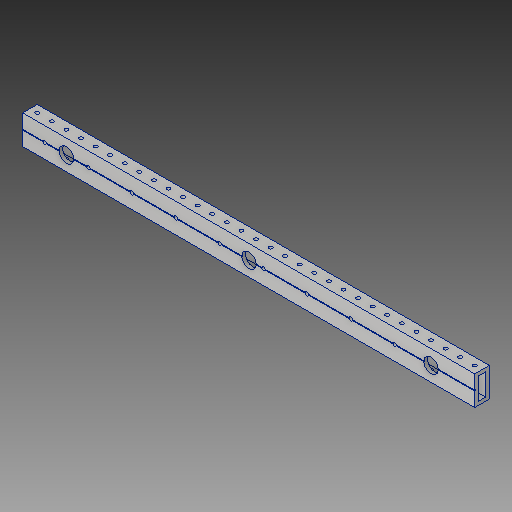
# Autodesk Inventor part: 2AM-17-01-Side Frame
Saved by Autodesk Inventor 2017 (Build 210142000, 142)
## iProperties
Created: 2017-12-28
Part Number: 2AM-17-01-Side Frame
Material: Aluminum 6061
Document SubType Name: Modeling
Designer: anikasoojin
Density: 2.7 g/cm^3
Appearance: Aluminum - Flat
Mass: 1616.08 g
Surface Area: 2052.62 cm^2
Volume: 598.55 cm^3
Author: anikasoojin
Autodesk Inventor part; units mm, degrees
ref_plane "YZ Plane" through (0, 0, 0) normal (1, 0, 0) x (0, 1, 0)
ref_plane "XZ Plane" through (0, 0, 0) normal (0, 1, 0) x (-1, 0, 0)
ref_plane "XY Plane" through (0, 0, 0) normal (0, 0, 1) x (1, 0, 0)
sketch "Sketch1" plane through (0, 0, 0) normal (1, 0, 0) x (0, 1, 0)
  line L0 (5.2493, 16.002) -> (-45.5507, 16.002)
  line L1 (-45.5507, 16.002) -> (-45.5507, -9.398)
  line L2 (-45.5507, -9.398) -> (5.2493, -9.398)
  line L3 (5.2493, -9.398) -> (5.2493, 16.002)
  line L4 (-1.1007, 9.652) -> (-39.2007, 9.652)
  line L5 (-39.2007, 9.652) -> (-39.2007, -3.048)
  line L6 (-39.2007, -3.048) -> (-1.1007, -3.048)
  line L7 (-1.1007, -3.048) -> (-1.1007, 9.652)
  point P0 (0, 0)
  dimension "d0" = 25.4
  dimension "d1" = 50.8
  dimension "d2" = 6.35
  constraints: 16 end point, 4 parallel, 2 perpendicular, 1 horizontal, 3 other
  measures "d0" distance of L2.end L0.start
  measures "d1" distance of L1.end L2.end
  measures "d2" distance between parallel lines of L3 L7
extrude "Extrusion1" add sketch "Sketch1" along normal blind 787.4
sketch "Sketch2" plane through (0, -45.5507, 16.002) normal (0, 0, 1) x (1, 0, 0)
  line L0 (0, 50.8) -> (0, 0) projected
  line L1 (0, 25.4) -> (787.4, 25.4) construction
  line L2 (787.4, 50.8) -> (787.4, 0) projected
  line L3 (0, 50.8) -> (787.4, 50.8) projected
  line L4 (393.7, 50.8) -> (394.6973, 0) construction
  line L5 (0, 0) -> (787.4, 0) projected
  circle A0 centre (394.1986, 25.4) radius 12.7
  circle A1 centre (711.2, 25.4) radius 12.7
  circle A2 centre (76.2, 25.4) radius 12.7
  circle A3 centre (38.1, 25.4) radius 3.175
  circle A4 centre (114.3, 25.4) radius 3.175
  circle A5 centre (190.5, 25.4) radius 3.175
  circle A6 centre (266.7, 25.4) radius 3.175
  circle A7 centre (342.9, 25.4) radius 3.175
  circle A8 centre (419.1, 25.4) radius 3.175
  circle A9 centre (495.3, 25.4) radius 3.175
  circle A10 centre (571.5, 25.4) radius 3.175
  circle A11 centre (647.7, 25.4) radius 3.175
  point P0 (0, 45.5507)
  dimension "d5" = 25.4
  dimension "d6" = 25.4
  dimension "d7" = 76.2
  dimension "d8" = 25.4
  dimension "d9" = 76.2
  dimension "d10" = 6.35
  dimension "d11" = 38.1
  dimension "d14" = 76.2
  constraints: 12 centre point, 4 end point, 4 midpoint, 4 point on line, 1 horizontal, 16 other
  measures "d5" diameter of A0
  measures "d6" diameter of A1
  measures "d7" distance of L1.end A1.centre
  measures "d8" diameter of A2
  measures "d9" distance of L1.start A2.centre
  measures "d10" diameter of A3
  measures "d11" distance of L1.start A3.centre
  measures "d14" distance of A3.centre A4.centre
extrude "Extrusion2" cut sketch "Sketch2" against normal through all contours A0 | A1 | A2 | A3 | A4 | A5 | A6 | A7 | A8 | A9 | A10 | A11
sketch "Sketch3" plane through (0, -45.5507, 16.002) normal (0, 0, 1) x (1, 0, 0)
  line L0 (0, 6.35) -> (0, 44.45) projected
  line L1 (0, 25.4) -> (787.4, 25.4) construction
  line L2 (787.4, 44.45) -> (787.4, 6.35) projected
  line L3 (0, 26.035) -> (787.4, 26.035)
  line L4 (0, 24.765) -> (787.4, 24.765)
  point P0 (0, 45.5507)
  dimension "d21" = 0.635
  dimension "d22" = 0.635
  constraints: 6 end point, 4 point on line, 2 midpoint, 2 parallel
  measures "d21" distance of L3.start L1.start
  measures "d22" distance of L1.start L4.start
extrude "Extrusion3" cut sketch "Sketch3" against normal blind 1.27
sketch "Sketch4" plane through (0, 5.2493, 16.002) normal (0, 1, 0) x (1, 0, 0)
  line L0 (0, 0) -> (0, 25.4) projected
  line L1 (30.4329, 12.7) -> (0, 12.7) construction
  circle A0 centre (12.7, 12.7) radius 3.175
  line L2 (55.8329, 12.7) -> (25.4, 12.7) construction
  circle A1 centre (38.1, 12.7) radius 3.175
  line L3 (81.2329, 12.7) -> (50.8, 12.7) construction
  circle A2 centre (63.5, 12.7) radius 3.175
  line L4 (106.6329, 12.7) -> (76.2, 12.7) construction
  circle A3 centre (88.9, 12.7) radius 3.175
  line L5 (132.0329, 12.7) -> (101.6, 12.7) construction
  circle A4 centre (114.3, 12.7) radius 3.175
  line L6 (157.4329, 12.7) -> (127, 12.7) construction
  circle A5 centre (139.7, 12.7) radius 3.175
  line L7 (182.8329, 12.7) -> (152.4, 12.7) construction
  circle A6 centre (165.1, 12.7) radius 3.175
  line L8 (208.2329, 12.7) -> (177.8, 12.7) construction
  circle A7 centre (190.5, 12.7) radius 3.175
  line L9 (233.6329, 12.7) -> (203.2, 12.7) construction
  circle A8 centre (215.9, 12.7) radius 3.175
  line L10 (259.0329, 12.7) -> (228.6, 12.7) construction
  circle A9 centre (241.3, 12.7) radius 3.175
  line L11 (284.4329, 12.7) -> (254, 12.7) construction
  circle A10 centre (266.7, 12.7) radius 3.175
  line L12 (309.8329, 12.7) -> (279.4, 12.7) construction
  circle A11 centre (292.1, 12.7) radius 3.175
  line L13 (335.2329, 12.7) -> (304.8, 12.7) construction
  circle A12 centre (317.5, 12.7) radius 3.175
  line L14 (360.6329, 12.7) -> (330.2, 12.7) construction
  circle A13 centre (342.9, 12.7) radius 3.175
  line L15 (386.0329, 12.7) -> (355.6, 12.7) construction
  circle A14 centre (368.3, 12.7) radius 3.175
  line L16 (411.4329, 12.7) -> (381, 12.7) construction
  circle A15 centre (393.7, 12.7) radius 3.175
  line L17 (436.8329, 12.7) -> (406.4, 12.7) construction
  circle A16 centre (419.1, 12.7) radius 3.175
  line L18 (462.2329, 12.7) -> (431.8, 12.7) construction
  circle A17 centre (444.5, 12.7) radius 3.175
  line L19 (487.6329, 12.7) -> (457.2, 12.7) construction
  circle A18 centre (469.9, 12.7) radius 3.175
  line L20 (513.0329, 12.7) -> (482.6, 12.7) construction
  circle A19 centre (495.3, 12.7) radius 3.175
  line L21 (538.4329, 12.7) -> (508, 12.7) construction
  circle A20 centre (520.7, 12.7) radius 3.175
  line L22 (563.8329, 12.7) -> (533.4, 12.7) construction
  circle A21 centre (546.1, 12.7) radius 3.175
  line L23 (589.2329, 12.7) -> (558.8, 12.7) construction
  circle A22 centre (571.5, 12.7) radius 3.175
  line L24 (614.6329, 12.7) -> (584.2, 12.7) construction
  circle A23 centre (596.9, 12.7) radius 3.175
  line L25 (640.0329, 12.7) -> (609.6, 12.7) construction
  circle A24 centre (622.3, 12.7) radius 3.175
  line L26 (665.4329, 12.7) -> (635, 12.7) construction
  circle A25 centre (647.7, 12.7) radius 3.175
  line L27 (690.8329, 12.7) -> (660.4, 12.7) construction
  circle A26 centre (673.1, 12.7) radius 3.175
  line L28 (716.2329, 12.7) -> (685.8, 12.7) construction
  circle A27 centre (698.5, 12.7) radius 3.175
  line L29 (741.6329, 12.7) -> (711.2, 12.7) construction
  circle A28 centre (723.9, 12.7) radius 3.175
  line L30 (767.0329, 12.7) -> (736.6, 12.7) construction
  circle A29 centre (749.3, 12.7) radius 3.175
  line L31 (792.4329, 12.7) -> (762, 12.7) construction
  circle A30 centre (774.7, 12.7) radius 3.175
  point P0 (0, 16.002)
  dimension "d25" = 6.35
  dimension "d26" = 12.7
  dimension "d29" = 25.4
  constraints: 62 end point, 31 centre point, 31 point on line, 2 horizontal, 1 collinear, 1 midpoint, 149 other
  measures "d25" diameter of A0
  measures "d26" distance from line of L0 A0.centre
  measures "d29" distance of L1.start L2.start
extrude "Extrusion4" cut sketch "Sketch4" against normal through all
body "Solid1"
